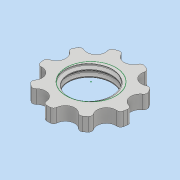
# Autodesk Inventor part: nakretka
Saved by Autodesk Inventor 2017 (Build 210142000, 142)
## iProperties
Created: 2017-11-03
Part Number: nakretka
Material: Ogólny
Document SubType Name: Modeling
Designer: Kuba01
Density: 1 g/cm^3
Appearance: Domyślna
Author: Kuba01
Autodesk Inventor part; units mm, degrees
ref_plane "YZ Plane" through (0, 0, 0) normal (1, 0, 0) x (0, 1, 0)
ref_plane "XZ Plane" through (0, 0, 0) normal (0, 1, 0) x (-1, 0, 0)
ref_plane "XY Plane" through (0, 0, 0) normal (0, 0, 1) x (1, 0, 0)
sketch "Szkic1" plane through (0, 0, 0) normal (0, 0, 1) x (1, 0, 0)
  circle A0 centre (0, 0) radius 14.5
  arc A1 (-5.4639, 24.3956) -> (5.4639, 24.3956) centre (0, 25) ccw
  arc A2 (-19.8668, 15.176) -> (-11.4956, 22.2003) centre (-16.0697, 19.1511) ccw
  arc A3 (-24.9738, -1.1447) -> (-23.0762, 9.6172) centre (-24.6202, 4.3412) ccw
  arc A4 (-18.3952, -16.9297) -> (-23.8592, -7.4659) centre (-21.6506, -12.5) ccw
  arc A5 (-3.2094, -24.7931) -> (-13.4782, -21.0556) centre (-8.5505, -23.4923) ccw
  arc A6 (13.4782, -21.0556) -> (3.2094, -24.7931) centre (8.5505, -23.4923) ccw
  arc A7 (23.8592, -7.4659) -> (18.3952, -16.9297) centre (21.6506, -12.5) ccw
  arc A8 (23.0762, 9.6172) -> (24.9738, -1.1447) centre (24.6202, 4.3412) ccw
  arc A9 (11.4956, 22.2003) -> (19.8668, 15.176) centre (16.0697, 19.1511) ccw
  arc A10 (11.4956, 22.2003) -> (5.4639, 24.3956) centre (0, 0) ccw
  arc A11 (23.0762, 9.6172) -> (19.8668, 15.176) centre (0, 0) ccw
  arc A12 (23.8592, -7.4659) -> (24.9738, -1.1447) centre (0, 0) ccw
  arc A13 (13.4782, -21.0556) -> (18.3952, -16.9297) centre (0, 0) ccw
  arc A14 (-3.2094, -24.7931) -> (3.2094, -24.7931) centre (0, 0) ccw
  arc A15 (-18.3952, -16.9297) -> (-13.4782, -21.0556) centre (0, 0) ccw
  arc A16 (-24.9738, -1.1447) -> (-23.8592, -7.4659) centre (0, 0) ccw
  arc A17 (-5.4639, 24.3956) -> (-11.4956, 22.2003) centre (0, 0) ccw
  arc A18 (-19.8668, 15.176) -> (-23.0762, 9.6172) centre (0, 0) ccw
  dimension "d0" = 29
  dimension "d4" = 360
  constraints: 36 point on circle, 19 centre point, 2 coincident, 37 other
  measures "d0" diameter of A0
extrude "Wyciągnięcie proste1" add sketch "Szkic1" along normal blind 8
fillet "Zaokrąglenie1" radius 2 18 edges at (3.2094, -24.7931, 4) (13.4782, -21.0556, 4) (18.3952, -16.9297, 4) (23.8592, -7.4659, 4) (24.9738, -1.1447, 4) (23.0762, 9.6172, 4) (19.8668, 15.176, 4) (11.4956, 22.2003, 4) (5.4639, 24.3956, 4) (-5.4639, 24.3956, 4) (-11.4956, 22.2003, 4) (-19.8668, 15.176, 4) (-23.0762, 9.6172, 4) (-24.9738, -1.1447, 4) (-23.8592, -7.4659, 4) (-18.3952, -16.9297, 4) (-3.2094, -24.7931, 4) (-13.4782, -21.0556, 4)
thread "Gwint1" size "M30x3.5" class "6H" standard "ANSI Metric M Profile" full length
sketch "Szkic2" plane through (0, 0, 8) normal (0, 0, 1) x (1, 0, 0)
  circle A0 centre (0, 0) radius 14.5 projected
sketch "Szkic4" plane through (0, 0, 8) normal (-1, 0, 0) x (0, 1, 0)
  line L0 (14.5, 0) -> (14.5, 8)
  line L1 (14.5, 8) -> (12.6056, 8)
  line L2 (12.6056, 8) -> (12.6056, 0)
  line L3 (12.6056, 0) -> (14.5, 0)
  line L4 (0, -6.0625) -> (0, 10.3437) projected
  constraints: 8 end point
revolve "Obrót1" add sketch "Szkic4" angle 360 about axis through (0, 0, 8) along (0, 0, -1) separate body
sketch "Szkic3" plane through (0, 14.5, 8) normal (1, 0, 0) x (0, 0, -1)
  line L0 (-1.75, 0.7578) -> (-2.3138, -0.2187) construction
  line L1 (-1.75, 0.7578) -> (-1.1862, -0.2187) construction
  line L2 (-1.75, 0.7578) -> (-1.75, 0) construction
  line L3 (-2.1875, 0) -> (-1.9349, 0) construction
  line L4 (0, -2.2733) -> (0.2187, -1.8944) construction
  line L5 (-3.5, -2.2733) -> (-3.7187, -1.8944) construction
  line L6 (-3.7187, -1.8944) -> (-3.5, -1.8944) construction
  line L7 (-3.2813, -1.8944) -> (-3.5, -2.2733) construction
  arc A0 (-1.9349, 0) -> (-2.3138, -0.2187) centre (-1.9349, -0.4375) ccw
  arc A1 (-1.1862, -0.2187) -> (-1.5651, 0) centre (-1.5651, -0.4375) ccw
  line L8 (0, -2.2733) -> (0, -1.8944) construction
  line L9 (-3.5, -2.2733) -> (-3.5, -1.8944) construction
  arc A2 (-0.2819, -1.7851) -> (-0.0925, -1.8944) centre (-0.0925, -1.6757) ccw
  line L10 (-1.1862, -0.2187) -> (-0.2819, -1.7851)
  line L11 (-1.9349, 0) -> (-1.5651, 0)
  line L12 (-2.3138, -0.2187) -> (-3.2181, -1.7851)
  line L13 (-0.0925, -1.8944) -> (0, -1.8944) construction
  line L14 (0, -1.8944) -> (0.2187, -1.8944) construction
  arc A3 (-3.4075, -1.8944) -> (-3.2181, -1.7851) centre (-3.4075, -1.6757) ccw
  line L15 (-3.2181, -1.7851) -> (-3.2813, -1.8944) construction
  line L16 (-3.5, -1.8944) -> (-3.4075, -1.8944) construction
  line L17 (-3.4075, -1.8944) -> (-0.0925, -1.8944)
  line L18 (0, 0) -> (0.4413, 0)
  line L19 (0, 0) -> (0, 0.419)
  line L20 (0, -2.2733) -> (-0.2819, -1.7851) construction
  dimension "d11" = 0.7578
  dimension "d12" = 0.4375
  dimension "d13" = 0.2188
  dimension "d14" = 0.3789
  dimension "d15" = 3.5
  dimension "Szkic3_MajorRadius" = 1.8944
  dimension "d17" = 60
  dimension "Szkic3_ThreadOffset" = 0
  dimension "Szkic3_MinorRadius" = 0
  constraints: 42 end point, 17 tangent, 8 point on circle, 6 parallel, 5 collinear, 4 centre point, 3 point on line, 3 vertical, 2 equal radius, 2 horizontal, 2 perpendicular, 1 equal length, 1 midpoint, 4 other
  measures "d11" distance from line of L0.start L3
  measures "d12" radius of A0
  measures "d13" radius of A2
  measures "d14" distance from line of L14 L4.start
  measures "d15" distance between parallel lines of L8 L9
  measures "Szkic3_MajorRadius" distance between parallel lines of L14 L18
  measures "d17" angle of L10 L12
  measures "Szkic3_ThreadOffset" distance between parallel lines of L19 L8
  measures "Szkic3_MinorRadius" distance between parallel lines of L18 L11
coil "Zwój1" sketch "Szkic3" operation cut axis through (0, 0, 8) along (0, 0, -1) pitch 3.5035 turns 4.281433 hand right bodies 2
equation "\"d11\" = 0.216506 * Szkic3_Pitch"
equation "\"d12\" = d20"
equation "\"d13\" = 0.0625 * Szkic3_Pitch"
equation "\"d14\" = 0.108253 * Szkic3_Pitch"
equation "\"d15\" = Szkic3_Pitch"
equation "\"d17\" = d22"
equation "\"d20\" = 0.125 * Szkic3_Pitch"
equation "\"Szkic3_Pitch\" = 3.5"
equation "\"d22\" = 60deg"
